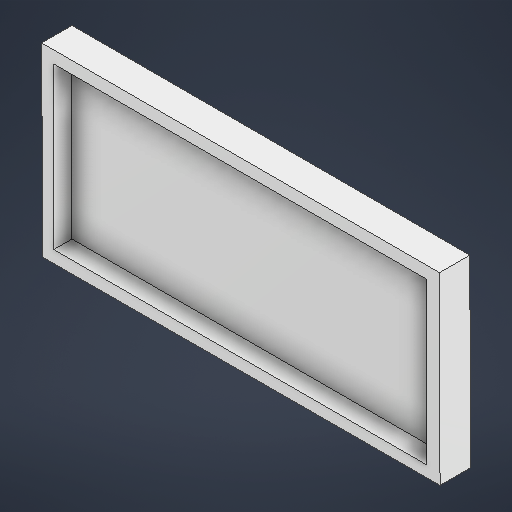
# Autodesk Inventor part: Deksel laser
Saved by Autodesk Inventor 2026.2 (Build 302298000, 298)
## iProperties
Created: 2026-05-05
Part Number: Deksel laser
Material: ABS Plastic
Document SubType Name: Modeling
Designer: Gameb
Density: 1.06 g/cm^3
Appearance: Smooth - White
Author: Gameb
Autodesk Inventor part; units mm, degrees
ref_plane "YZ Plane" through (0, 0, 0) normal (1, 0, 0) x (0, 1, 0)
ref_plane "XZ Plane" through (0, 0, 0) normal (0, 1, 0) x (-1, 0, 0)
ref_plane "XY Plane" through (0, 0, 0) normal (0, 0, 1) x (1, 0, 0)
sketch "Sketch1" plane through (0, 0, 0) normal (0, 0, 1) x (1, 0, 0)
  line L0 (-56.6552, 0) -> (-56.6552, 8.2905)
  line L1 (-56.6552, 0) -> (-56.6552, 26.5)
  line L2 (-56.6552, 26.5) -> (-56.6552, -26.5)
  line L3 (-56.6552, -26.5) -> (66.3448, -26.5)
  line L4 (66.3448, -26.5) -> (66.3448, 26.5)
  line L5 (66.3448, 26.5) -> (-56.6552, 26.5)
  line L6 (-60.3103, -26.5) -> (-60.3103, -30.1552)
  line L7 (56.6552, -30.1552) -> (60.3103, -30.1552)
  line L8 (-56.6552, 30.5) -> (-60.6552, 30.5)
  line L9 (-60.6552, 30.5) -> (-60.3103, -30.499)
  line L10 (-60.3103, -30.499) -> (70.6892, -30.1552)
  line L11 (70.6892, -30.1552) -> (70.53, 30.5)
  line L12 (70.53, 30.5) -> (-60.6552, 30.5)
  point P0 (0, 0)
  dimension "d19" = 123
  dimension "d20" = 53
  constraints: 26 end point, 5 perpendicular, 4 point on line, 1 collinear
  measures "d19" distance of L4.end L1.end
  measures "d20" distance of L1.end L2.end
extrude "Extrusion1" add sketch "Sketch1" against normal blind 4 contours L0 L1 L5 L4 L3 L2 | L12 L11 L10 L9 L8
extrude "Extrusion2" add sketch "Sketch1" along normal blind 6
body "Solid1"
